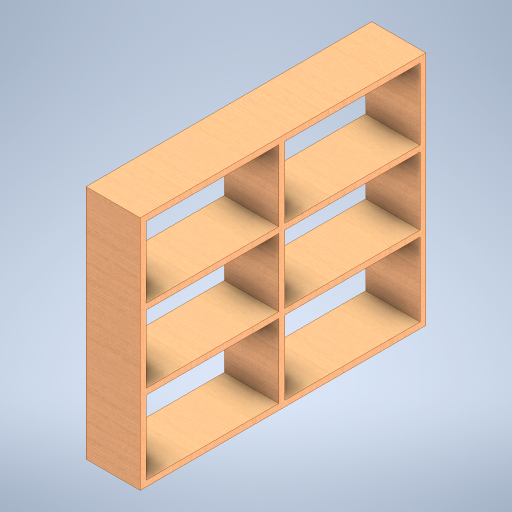
# Autodesk Inventor part: Estanteria
Saved by Autodesk Inventor 2023 (Build 270158000, 158)
## iProperties
Created: 2023-06-19
Part Number: Estanteria
Material: Wood (Cherry)
Document SubType Name: Modeling
Designer: Usuario
Density: 0.63 g/cm^3
Appearance: Cherry - Natural Low Gloss
Author: Usuario
Autodesk Inventor part; units mm, degrees
ref_plane "YZ Plane" through (0, 0, 0) normal (1, 0, 0) x (0, 1, 0)
ref_plane "XZ Plane" through (0, 0, 0) normal (0, 1, 0) x (-1, 0, 0)
ref_plane "XY Plane" through (0, 0, 0) normal (0, 0, 1) x (1, 0, 0)
sketch "Sketch1" plane through (0, 0, 0) normal (1, 0, 0) x (0, 1, 0)
  line L0 (345.6873, 423.9836) -> (-90.3127, 423.9836)
  line L1 (-90.3127, 423.9836) -> (-90.3127, -104.0164)
  line L2 (-90.3127, -104.0164) -> (345.6873, -104.0164)
  line L3 (345.6873, -104.0164) -> (345.6873, 423.9836)
  line L4 (334.6873, -93.0164) -> (334.6873, 156.9836)
  line L5 (334.6873, 167.9836) -> (334.6873, 412.9836)
  line L6 (203.6873, 412.9836) -> (203.6873, 167.9836)
  line L7 (203.6873, 156.9836) -> (203.6873, -93.0164)
  line L8 (192.6873, 412.9836) -> (192.6873, 167.9836)
  line L9 (192.6873, 156.9836) -> (192.6873, -93.0164)
  line L10 (334.6873, 156.9836) -> (203.6873, 156.9836)
  line L11 (334.6873, 167.9836) -> (203.6873, 167.9836)
  line L12 (334.6873, 412.9836) -> (203.6873, 412.9836)
  line L13 (192.6873, 412.9836) -> (67.6873, 412.9836)
  line L14 (56.6873, 412.9836) -> (-79.3127, 412.9836)
  line L15 (192.6873, 156.9836) -> (67.6873, 156.9836)
  line L16 (56.6873, 156.9836) -> (-79.3127, 156.9836)
  line L17 (192.6873, 167.9836) -> (67.6873, 167.9836)
  line L18 (56.6873, 167.9836) -> (-79.3127, 167.9836)
  line L19 (56.6873, 412.9836) -> (56.6873, 167.9836)
  line L20 (56.6873, 156.9836) -> (56.6873, -93.0164)
  line L21 (67.6873, 412.9836) -> (67.6873, 167.9836)
  line L22 (67.6873, 156.9836) -> (67.6873, -93.0164)
  line L23 (-79.3127, -93.0164) -> (56.6873, -93.0164)
  line L24 (67.6873, -93.0164) -> (192.6873, -93.0164)
  line L25 (203.6873, -93.0164) -> (334.6873, -93.0164)
  line L26 (-79.3127, 412.9836) -> (-79.3127, 167.9836)
  line L27 (-79.3127, 156.9836) -> (-79.3127, -93.0164)
  constraints: 56 end point, 43 perpendicular, 15 parallel, 4 horizontal
extrude "Extrusion1" add sketch "Sketch1" against normal blind 100
body "Solid1"
